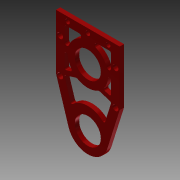
# Autodesk Inventor part: Swerve Wheel + Carriage Outline V1
Saved by Autodesk Inventor 2013 (Build 170138000, 138)
## iProperties
Created: 2013-04-01
Part Number: Swerve Wheel + Carriage Outline V1
Material: Generic
Document SubType Name: Sheet Metal
Designer: mvarma
Density: 1 g/cm^3
Sheet Metal Rule: Default
Author: mvarma
Autodesk Inventor part; units mm, degrees
ref_plane "YZ Plane" through (0, 0, 0) normal (1, 0, 0) x (0, 1, 0)
ref_plane "XZ Plane" through (0, 0, 0) normal (0, 1, 0) x (-1, 0, 0)
ref_plane "XY Plane" through (0, 0, 0) normal (0, 0, 1) x (1, 0, 0)
sketch "Sketch1" plane through (0, 0, 0) normal (0, 0, 1) x (1, 0, 0)
  circle A0 centre (0, 0) radius 38.1 construction
  circle A1 centre (0, 0) radius 41.275 construction
  line L0 (-7.3323, 0) -> (-3.6662, 6.35) construction
  line L1 (-3.6662, 6.35) -> (3.6662, 6.35) construction
  line L2 (3.6662, 6.35) -> (7.3323, 0) construction
  line L3 (7.3323, 0) -> (3.6662, -6.35) construction
  line L4 (3.6662, -6.35) -> (-3.6662, -6.35) construction
  line L5 (-3.6662, -6.35) -> (-7.3323, 0) construction
  circle A2 centre (0, 0) radius 14.2875
  circle A3 centre (0, 0) radius 15.875 construction
  circle A4 centre (0, 0) radius 8.7313 construction
  circle A5 centre (0, 0) radius 22.225
  line L6 (34.925, 37.2364) -> (34.925, 97.5614)
  line L7 (34.925, 97.5614) -> (-34.925, 97.5614)
  line L8 (-34.925, 97.5614) -> (-34.925, 37.2364)
  line L9 (34.925, 37.2364) -> (-34.925, 37.2364) construction
  line L10 (34.925, 37.2364) -> (21.2128, -6.6308)
  line L11 (-34.925, 37.2364) -> (-21.2128, -6.6308)
  circle A6 centre (-30.353, 37.2364) radius 3.9624 construction
  line L12 (53.34, 97.5614) -> (-53.34, 97.5614) construction
  line L13 (-53.34, 97.5614) -> (-53.34, 107.0864) construction
  line L14 (-53.34, 107.0864) -> (53.34, 107.0864) construction
  line L15 (53.34, 107.0864) -> (53.34, 97.5614) construction
  circle A7 centre (-222.5199, 24.1494) radius 53.34 construction
  line L16 (-190.7699, 59.0744) -> (-254.2699, 59.0744) construction
  line L17 (-254.2699, 59.0744) -> (-254.2699, -10.7756) construction
  line L18 (-254.2699, -10.7756) -> (-190.7699, -10.7756) construction
  line L19 (-190.7699, -10.7756) -> (-190.7699, 59.0744) construction
  line L20 (-195.5324, 59.0744) -> (-195.5324, -10.7756) construction
  line L21 (-249.5074, 59.0744) -> (-249.5074, -10.7756) construction
  line L22 (-209.8199, 68.5994) -> (-235.2199, 68.5994) construction
  line L23 (-235.2199, 68.5994) -> (-235.2199, -20.3006) construction
  line L24 (-235.2199, -20.3006) -> (-209.8199, -20.3006) construction
  line L25 (-209.8199, -20.3006) -> (-209.8199, 68.5994) construction
  line L26 (34.925, 88.0364) -> (-34.925, 88.0364) construction
  circle A8 centre (30.353, 37.2364) radius 3.9624 construction
  circle A9 centre (30.353, 75.3364) radius 3.9624 construction
  circle A10 centre (-30.353, 75.3364) radius 3.9624 construction
  line L27 (34.925, 92.7989) -> (-34.925, 92.7989) construction
  circle A11 centre (0, 63.0333) radius 14.2875
  circle A12 centre (0, 63.0333) radius 15.875 construction
  line L28 (7.3323, 63.0333) -> (3.6662, 56.6833) construction
  line L29 (3.6662, 56.6833) -> (-3.6662, 56.6833) construction
  line L30 (-3.6662, 56.6833) -> (-7.3323, 63.0333) construction
  line L31 (-7.3323, 63.0333) -> (-3.6662, 69.3833) construction
  line L32 (-3.6662, 69.3833) -> (3.6662, 69.3833) construction
  line L33 (3.6662, 69.3833) -> (7.3323, 63.0333) construction
  point P0 (22.225, 92.7989)
  point P1 (0, 92.7989)
  point P2 (-22.225, 92.7989)
  dimension "d0" = 76.2
  dimension "d2" = 82.55
  dimension "d3" = 12.7
  dimension "d4" = 28.575
  dimension "d5" = 31.75
  dimension "d6" = 17.4625
  dimension "d7" = 44.45
  dimension "d8" = 69.85
  dimension "d9" = 34.925
  dimension "d10" = 37.2364
  dimension "d13" = 7.9248
  dimension "d14" = 9.525
  dimension "d15" = 106.68
  dimension "d16" = 53.34
  dimension "d17" = 106.68
  dimension "d18" = 69.85
  dimension "d19" = 34.925
  dimension "d20" = 63.5
  dimension "d21" = 31.75
  dimension "d22" = 4.7625
  dimension "d23" = 4.7625
  dimension "d24" = 25.4
  dimension "d25" = 14.2875
  dimension "d26" = 88.9
  dimension "d27" = 14.2875
  dimension "d28" = 44.45
  dimension "d29" = 4.572
  dimension "d30" = 9.525
  dimension "d31" = 0
  dimension "d32" = 7.9248
  dimension "d33" = 4.572
  dimension "d34" = 7.9248
  dimension "d35" = 7.9248
  dimension "d36" = 4.572
  dimension "d37" = 4.572
  dimension "d38" = 38.1
  dimension "d39" = 38.1
  dimension "d44" = 4.7625
  dimension "d45" = 34.925
  dimension "d46" = 12.7
  dimension "d47" = 12.7
  dimension "d48" = 28.575
  dimension "d52" = 31.75
  dimension "d53" = 12.7
  dimension "d54" = 25.0031
  dimension "d72" = 50.8
  dimension "d73" = 34.925
  constraints: 68 end point, 13 centre point, 13 coincident, 12 point on line, 10 perpendicular, 7 parallel, 5 horizontal, 2 point on circle, 2 tangent, 1 midpoint, 27 other
  measures "d0" diameter of A0
  measures "d2" diameter of A1
  measures "d3" distance between parallel lines of L4 L1
  measures "d4" diameter of A2
  measures "d5" diameter of A3
  measures "d6" diameter of A4
  measures "d7" diameter of A5
  measures "d8" distance between parallel lines of L8 L6
  measures "d9" distance from line of point (0, 0) L8
  measures "d10" distance from line of L9 point (0, 0)
  measures "d13" diameter of A6
  measures "d14" distance of L14.end L12.start
  measures "d15" distance of L13.end L14.end
  measures "d16" horizontal distance of L12.start point (0, 0)
  measures "d17" diameter of A7
  measures "d18" distance of L18.end L16.start
  measures "d19" distance from line of A7.centre L18
  measures "d20" distance of L17.end L18.end
  measures "d21" distance from line of L19 A7.centre
  measures "d22" distance between parallel lines of L17 L21
  measures "d23" distance between parallel lines of L19 L20
  measures "d24" distance between parallel lines of L23 L25
  measures "d25" distance between parallel lines of L20 L25
  measures "d26" distance of L22.end L23.end
  measures "d27" distance between parallel lines of L21 L23
  measures "d28" distance from line of A7.centre L24
  measures "d29" distance from line of L8 A6.centre
  measures "d30" distance between parallel lines of L7 L26
  measures "d31" distance between parallel lines of L7 L12
  measures "d32" diameter of A8
  measures "d33" distance from line of L6 A8.centre
  measures "d34" diameter of A9
  measures "d35" diameter of A10
  measures "d36" distance from line of L8 A10.centre
  measures "d37" distance from line of L6 A9.centre
  measures "d38" distance from line of L9 A10.centre
  measures "d39" distance from line of L9 A9.centre
  measures "d44" distance between parallel lines of L26 L27
  measures "d45" distance from line of L8 point (0, 92.799)
  measures "d46" distance from line of L8 point (-22.225, 92.799)
  measures "d47" distance from line of L6 point (22.225, 92.799)
  measures "d48" diameter of A11
  measures "d52" diameter of A12
  measures "d53" distance between parallel lines of L29 L32
  measures "d54" distance from line of L26 A12.centre
  measures "d72" distance between parallel lines of L9 L26
  measures "d73" distance from line of L8 A11.centre
extrude "Plate1" add sketch "Sketch1" along normal blind 4.7625 contours A2 | A5 | A5 L11 L8 L7 L6 L10 | A11
extrude "Cut1" cut sketch "Sketch1" along normal up to next contours A2 | A11
hole "Hole1" at (30.353, 75.3364, 0) at (30.353, 37.2364, 0) at (-30.353, 37.2364, 0) at (-30.353, 75.3364, 0) direction (0, 0, 1) diameter 6.35 end through all
hole "Hole2" at (22.225, 92.7989, 0) at (0, 92.7989, 0) at (-22.225, 92.7989, 0) direction (0, 0, 1) diameter 4.9784 end through all clearance for "Socket Head Cap Screw" size "#10" standard "Ansi Unified Screw Threads"
sketch "Sketch2" plane through (0, 0, 0) normal (0, 0, -1) x (-1, 0, 0)
  line L0 (-24.3186, 40.5518) -> (-13.4446, 43.9508)
  line L1 (24.3186, 40.5518) -> (13.4446, 43.9508)
  line L2 (-25.3602, 38.563) -> (-18.9359, 18.0109)
  line L3 (18.9359, 18.0109) -> (25.3602, 38.563)
  arc A0 (16.3319, 17.3293) -> (-16.3319, 17.3293) centre (0, 0) ccw
  arc A1 (-1.0222, 40.8318) -> (10.9351, 43.6845) centre (0, 63.0333) ccw
  arc A2 (-24.3186, 40.5518) -> (-25.3602, 38.563) centre (-23.845, 39.0366) ccw
  arc A3 (25.3602, 38.563) -> (24.3186, 40.5518) centre (23.845, 39.0366) ccw
  arc A4 (-18.9359, 18.0109) -> (-16.3319, 17.3293) centre (-17.4207, 18.4845) ccw
  arc A5 (-10.9351, 43.6845) -> (-1.0222, 40.8318) centre (0, 63.0333) ccw
  arc A6 (17.8398, 49.7784) -> (22.1389, 61.0785) centre (0, 63.0333) ccw
  arc A7 (-10.9351, 43.6845) -> (-13.4446, 43.9508) centre (-12.4973, 40.9204) ccw
  arc A8 (13.4446, 43.9508) -> (10.9351, 43.6845) centre (12.4973, 40.9204) ccw
  line L4 (-25.3602, 38.563) -> (-25.8338, 40.0782) construction
  line L5 (-24.3186, 40.5518) -> (-25.8338, 40.0782) construction
  line L6 (-23.3389, 45.8478) -> (-18.6405, 47.3164)
  line L7 (18.6405, 47.3164) -> (23.3389, 45.8478)
  line L8 (-25.4, 47.363) -> (-25.4, 61.0785)
  line L9 (25.4, 47.363) -> (25.4, 61.0785)
  line L10 (-25.4, 61.0785) -> (-22.1389, 61.0785) construction
  line L11 (25.4, 61.0785) -> (22.1389, 61.0785) construction
  arc A9 (-22.1389, 61.0785) -> (-25.4, 61.0785) centre (-23.7694, 61.0785) ccw
  arc A10 (25.4, 61.0785) -> (22.1389, 61.0785) centre (23.7694, 61.0785) ccw
  arc A11 (-25.4, 47.363) -> (-23.3389, 45.8478) centre (-23.8125, 47.363) ccw
  arc A12 (-18.6405, 47.3164) -> (-17.8398, 49.7784) centre (-19.1141, 48.8316) ccw
  arc A13 (17.8398, 49.7784) -> (18.6405, 47.3164) centre (19.1141, 48.8316) ccw
  arc A14 (23.3389, 45.8478) -> (25.4, 47.363) centre (23.8125, 47.363) ccw
  arc A15 (-22.1389, 61.0785) -> (-17.8398, 49.7784) centre (0, 63.0333) ccw
  arc A16 (22.1389, 61.0785) -> (20.7911, 70.8869) centre (0, 63.0333) ccw
  line L12 (-25.4, 61.0785) -> (-25.4, 86.4489)
  line L13 (-23.8125, 88.0364) -> (23.8125, 88.0364)
  line L14 (25.4, 86.4489) -> (25.4, 61.0785)
  arc A17 (-25.4, 71.7284) -> (-20.7911, 70.8869) centre (-23.0187, 71.7284) ccw
  arc A18 (-8.744, 83.4659) -> (-9.6808, 88.0364) centre (-9.6808, 85.6552) ccw
  arc A19 (9.6808, 88.0364) -> (8.744, 83.4659) centre (9.6808, 85.6552) ccw
  arc A20 (20.7911, 70.8869) -> (25.4, 71.7284) centre (23.0188, 71.7284) ccw
  arc A21 (-9.6808, 88.0364) -> (-8.744, 83.4659) centre (-9.6808, 85.6552) ccw
  arc A22 (-20.7911, 70.8869) -> (-25.4, 71.7284) centre (-23.0187, 71.7284) ccw
  arc A23 (8.744, 83.4659) -> (9.6808, 88.0364) centre (9.6808, 85.6552) ccw
  arc A24 (25.4, 71.7284) -> (20.7911, 70.8869) centre (23.0188, 71.7284) ccw
  arc A25 (20.7911, 70.8869) -> (8.744, 83.4659) centre (0, 63.0333) ccw
  arc A26 (8.744, 83.4659) -> (-8.744, 83.4659) centre (0, 63.0333) ccw
  arc A27 (-8.744, 83.4659) -> (-20.7911, 70.8869) centre (0, 63.0333) ccw
  arc A28 (-20.7911, 70.8869) -> (-22.1389, 61.0785) centre (0, 63.0333) ccw
  arc A29 (-23.8125, 88.0364) -> (-25.4, 86.4489) centre (-23.8125, 86.4489) ccw
  arc A30 (25.4, 86.4489) -> (23.8125, 88.0364) centre (23.8125, 86.4489) ccw
  circle A31 centre (0, 92.7989) radius 2.4892 projected
  circle A32 centre (-22.225, 92.7989) radius 2.4892 projected
  circle A33 centre (22.225, 92.7989) radius 2.4892 projected
  circle A34 centre (30.353, 37.2364) radius 3.175 projected
  circle A35 centre (-30.353, 75.3364) radius 3.175 projected
  circle A36 centre (-30.353, 37.2364) radius 3.175 projected
  circle A37 centre (30.353, 75.3364) radius 3.175 projected
  circle A38 centre (0, 0) radius 14.2875 projected
  circle A39 centre (0, 63.0333) radius 14.2875 projected
  arc A40 (-21.2128, -6.6308) -> (21.2128, -6.6308) centre (0, 0) ccw projected
  line L15 (34.925, 37.2364) -> (21.2128, -6.6308) projected
  line L16 (34.925, 97.5614) -> (34.925, 37.2364) projected
  line L17 (-34.925, 97.5614) -> (34.925, 97.5614) projected
  line L18 (-34.925, 37.2364) -> (-34.925, 97.5614) projected
  line L19 (-21.2128, -6.6308) -> (-34.925, 37.2364) projected
  line L20 (-25.8338, 40.0782) -> (-34.925, 37.2364) construction
  line L21 (24.3186, 40.5518) -> (34.925, 37.2364) construction
  arc A41 (16.3319, 17.3293) -> (18.9359, 18.0109) centre (17.4207, 18.4845) ccw
  point P0 (18.1313, 15.4367)
  point P1 (-25.4, 45.2035)
  point P2 (25.4, 45.2035)
  dimension "d79" = 1.5875
  dimension "d80" = 1.5875
  dimension "d81" = 3.175
  dimension "d84" = 4.7625
  dimension "d85" = 15.875
  dimension "d86" = 15.875
  dimension "d87" = 1.5875
  dimension "d89" = 4.7625
  dimension "d91" = 4.7625
  dimension "d92" = 1.5875
  dimension "d93" = 9.525
  dimension "d94" = 9.525
  dimension "d95" = 9.525
  dimension "d96" = 9.525
  dimension "d97" = 9.525
  dimension "d98" = 22.225
  dimension "d99" = 22.225
  dimension "d104" = 10.6064
  dimension "d106" = 35.9472
  dimension "d107" = 23.8125
  dimension "d108" = 1.5875
  constraints: 73 point on circle, 36 tangent, 34 end point, 32 centre point, 10 point on line, 9 equal radius, 9 perpendicular, 3 parallel, 2 coincident, 2 collinear, 2 midpoint
  measures "d79" radius of A2
  measures "d80" radius of A4
  measures "d81" radius of A7
  measures "d84" distance between parallel lines of L6 L0
  measures "d85" distance of point (-25.4, 45.204) L8.end
  measures "d86" distance of point (25.4, 45.204) L9.end
  measures "d87" radius of A11
  measures "d89" distance between parallel lines of L1 L7
  measures "d91" diameter of A20
  measures "d92" radius of A29
  measures "d93" distance between parallel lines of L17 L13
  measures "d94" distance between parallel lines of L18 L12
  measures "d95" distance between parallel lines of L16 L14
  measures "d96" distance between parallel lines of L15 L3
  measures "d97" distance between parallel lines of L19 L2
  measures "d98" radius of A5
  measures "d99" radius of A15
  measures "d104" distance from line of L21.start L16
  measures "d106" distance from line of A1.start L16
  measures "d107" radius of A0
  measures "d108" radius of A41
extrude "Cut2" cut sketch "Sketch2" against normal blind 4.7625 contours L0 A7 A5 A1 A8 L1 A3 L3 A41 A0 A4 L2 A2 | A6 A16 A10 L9 A14 L7 A13 | A10 A16 | A24 A20 | A25 A23 L13 A30 L14 A24 | A19 A23 | A21 A18 | A27 A22 L12 A29 L13 A21 | A17 A22 | A28 A15 A12 L6 A11 L8 A9 | A9 A28
equation "\"d9\" = 0.5 * d8"
equation "\"d16\" = 0.5 * d15"
equation "\"d19\" = 0.5 * d18"
equation "\"d21\" = 0.5 * d20"
equation "\"d22\" = d23"
equation "\"d25\" = d27"
equation "\"d28\" = 0.5 * d26"
equation "\"d32\" = d13"
equation "\"d33\" = d29"
equation "\"d34\" = d32"
equation "\"d35\" = d13"
equation "\"d36\" = d29"
equation "\"d37\" = d29"
equation "\"d39\" = d38"
equation "\"d44\" = 0.5 * d30"
equation "\"d45\" = d42"
equation "\"d47\" = d46"
equation "\"d56\" = Thickness"
equation "\"d63\" = Thickness"
equation "\"d70\" = Thickness"
equation "\"d79\" = d80"
equation "\"BendRadius\" = Thickness"
equation "\"BendReliefWidth\" = Thickness"
equation "\"BendReliefDepth\" = 0.5 * Thickness"
equation "\"CornerReliefSize\" = 4 * Thickness"
equation "\"MinimumRemnant\" = 2 * Thickness"
equation "\"TransitionRadius\" = BendRadius"
equation "\"JacobiRadiusSize\" = Thickness"
equation "\"GapSize\" = Thickness"
equation "\"d55\" = BendRadius"
equation "\"Thickness\" = 4.7625"
equation "\"d42\" = 34.925"
body "Solid1"
